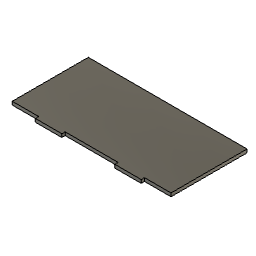
front (Autodesk Fusion 360 design; units mm, degrees)
Autodesk Fusion 360 part; units mm, degrees
sketch "Sketch1" plane through (0, 0, 0) normal (0, 0, 1) x (1, 0, 0)
  line L0 (-76.2, 38.1) -> (76.2, 38.1)
  line L1 (76.2, 38.1) -> (76.2, -38.1)
  line L2 (76.2, -38.1) -> (-76.2, -38.1)
  line L3 (-76.2, -38.1) -> (-76.2, 38.1)
  dimension "d1" = 152.4
  dimension "d2" = 76.2
  dimension "d3" = 76.2
  dimension "d4" = 38.1
  constraint horizontal L0
  constraint vertical L1
  constraint horizontal L2
  constraint vertical L3
  measures "d1" distance of L0.start L0.end
  measures "d2" distance of L0.start L2.end
  measures "d3" horizontal distance of origin L0.start
  measures "d4" vertical distance of origin L0.start
extrude "Extrude1" add sketch "Sketch1" along normal blind 3.175
sketch "Sketch2" plane through (0, 0, 3.175) normal (0, 0, 1) x (-1, 0, 0)
  line L0 (76.2, 38.1) -> (-76.2, 38.1)
  line L1 (-76.2, 38.1) -> (-76.2, -38.1)
  line L2 (-76.2, -38.1) -> (76.2, -38.1)
  line L3 (76.2, -38.1) -> (76.2, 38.1)
  line L4 (76.2, 38.1) -> (50.8, 38.1)
  line L5 (50.8, 38.1) -> (50.8, 34.925)
  line L6 (50.8, 34.925) -> (76.2, 34.925)
  line L7 (76.2, 34.925) -> (76.2, 38.1)
  line L8 (-76.2, 38.1) -> (-50.8, 38.1)
  line L9 (-50.8, 38.1) -> (-50.8, 34.925)
  line L10 (-50.8, 34.925) -> (-76.2, 34.925)
  line L11 (-76.2, 34.925) -> (-76.2, 38.1)
  line L12 (25.4, 38.1) -> (-25.4, 38.1)
  line L13 (-25.4, 38.1) -> (-25.4, 34.925)
  line L14 (-25.4, 34.925) -> (25.4, 34.925)
  line L15 (25.4, 34.925) -> (25.4, 38.1)
  dimension "d7" = 25.4
  dimension "d8" = 3.175
  dimension "d9" = 25.4
  dimension "d10" = 3.175
  dimension "d11" = 25.4
  dimension "d12" = 25.4
  dimension "d13" = 3.175
  constraint horizontal L4
  constraint vertical L5
  constraint horizontal L6
  constraint vertical L7
  constraint coincident L0.start L3.end
  constraint horizontal L8
  constraint vertical L9
  constraint horizontal L10
  constraint vertical L11
  constraint coincident L0.end L1.start
  constraint horizontal L12
  constraint vertical L13
  constraint horizontal L14
  constraint vertical L15
  constraint coincident L0 L12.start
  measures "d7" distance of L0.start L4.end
  measures "d8" distance of L0.start L6.end
  measures "d9" distance of L0.end L8.end
  measures "d10" distance of L0.end L10.end
  measures "d11" distance of L8.end L12.end
  measures "d12" distance of L4.end L12.start
  measures "d13" distance of L12.start L14.end
extrude "Extrude2" cut sketch "Sketch2" against normal through all contours L0 L3 L4 L5 L6 L7 | L0 L12 L13 L14 L15 | L0 L1 L8 L9 L10 L11
